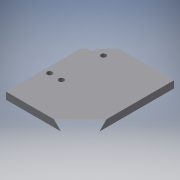
# Autodesk Inventor part: Internal support motor-ball bracket
Saved by Autodesk Inventor 2016 (Build 200138000, 138)
## iProperties
Created: 2017-06-06
Part Number: Internal support motor-ball bracket
Material: Generic
Document SubType Name: Modeling
Designer: m228540
Density: 1 g/cm^3
Appearance: Default
Author: m228540
Autodesk Inventor part; units mm, degrees
ref_plane "YZ Plane" through (0, 0, 0) normal (1, 0, 0) x (0, 1, 0)
ref_plane "XZ Plane" through (0, 0, 0) normal (0, 1, 0) x (-1, 0, 0)
ref_plane "XY Plane" through (0, 0, 0) normal (0, 0, 1) x (1, 0, 0)
sketch "Sketch1" plane through (0, 0, 0) normal (0, 0, 1) x (1, 0, 0)
  line L0 (-28.6614, -59.685) -> (66.3386, -59.685)
  line L1 (66.3386, -59.685) -> (66.3386, 60.315)
  line L2 (66.3386, 60.315) -> (-28.6614, 60.315)
  line L3 (-28.6614, 60.315) -> (-28.6614, -59.685)
  point P0 (0, 0)
  dimension "d0" = 120
  dimension "d1" = 95
  constraints: 8 end point, 2 parallel, 1 horizontal, 1 perpendicular
  measures "d0" distance of L2.end L0.start
  measures "d1" distance of L1.end L2.end
extrude "Extrusion1" add sketch "Sketch1" along normal blind 6
sketch "Sketch3" plane through (0, 0, 0) normal (0, 0, -1) x (-1, 0, 0)
  line L0 (-66.3386, 60.315) -> (28.6614, 60.315) projected
  line L1 (28.6614, 60.315) -> (28.6614, 53.315)
  line L2 (28.6614, 60.315) -> (28.6614, -59.685) projected
  line L3 (28.6614, 53.315) -> (-6.3386, 53.315)
  line L4 (-6.3386, 53.315) -> (-6.3386, -21.685)
  line L5 (-6.3386, -21.685) -> (28.6614, -21.685)
  line L6 (28.6614, -21.685) -> (28.6614, -59.685)
  line L7 (28.6614, -59.685) -> (-66.3386, -59.685) projected
  line L8 (28.6614, -59.685) -> (-66.3386, -59.685)
  line L9 (-66.3386, -59.685) -> (-66.3386, 60.315) projected
  line L10 (-66.3386, -59.685) -> (-66.3386, 60.315)
  line L11 (-66.3386, 60.315) -> (28.6614, 60.315)
  point P0 (0, 0)
  dimension "d9" = 7
  dimension "d10" = 35
  dimension "d11" = 75
  constraints: 16 end point, 4 collinear, 2 perpendicular, 2 point on line, 1 horizontal
  measures "d9" distance of L0.end L1.end
  measures "d10" distance of L1.end L3.end
  measures "d11" distance of L3.end L4.end
extrude "Extrusion3" add sketch "Sketch3" along normal blind 3 contours L0 L1 L3 L4 L5 L2 L7 L9
fillet "Fillet1" radius 7 2 edges at (6.3386, -21.685, -1.5) (6.3386, 53.315, -1.5)
sketch "Sketch4" plane through (0, 0, 0) normal (0, 0, -1) x (-1, 0, 0)
  circle A0 centre (14.6614, 40.6422) radius 5.5 projected
  circle A1 centre (21.1614, 38.2493) radius 3.3 projected
  circle A2 centre (21.1614, -15.7507) radius 3.3 projected
  circle A3 centre (14.6614, -19.3578) radius 5.5 projected
  point P0 (0, 0)
extrude "Extrusion4" cut sketch "Sketch4" against normal through all
body "Solid1"
